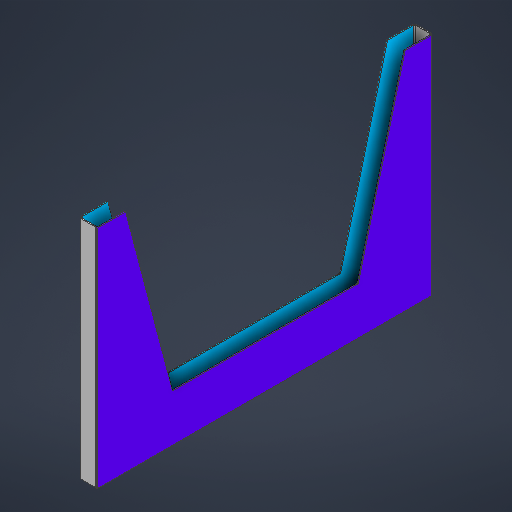
# Autodesk Inventor part: Div_Big
Saved by Autodesk Inventor 2025.1 (Build 291241000, 241)
## iProperties
Created: 2024-09-26
Part Number: Div_Big
Material: Generic
Document SubType Name: Sheet Metal
Designer: rocky
Density: 1 g/cm^3
Sheet Metal Rule: Default
Appearance: Default
Flat Pattern Width: 60.96 cm
Flat Pattern Length: 189.571 cm
Flat Pattern Area: 11556.3 cm^2
Sheet Metal Width: 24.000 in
Sheet Metal Length: 74.634 in
Sheet Metal Area: 1791.223 in^2
Author: rocky
Autodesk Inventor part; units mm, degrees
ref_plane "YZ Plane" through (0, 0, 0) normal (1, 0, 0) x (0, 1, 0)
ref_plane "XZ Plane" through (0, 0, 0) normal (0, 1, 0) x (-1, 0, 0)
ref_plane "XY Plane" through (0, 0, 0) normal (0, 0, 1) x (1, 0, 0)
sketch "Sketch1" plane through (0, 0, 0) normal (1, 0, 0) x (0, 1, 0)
  line L0 (0, 0) -> (609.6, 0)
  line L1 (609.6, 0) -> (609.6, -908.05)
  line L2 (609.6, -908.05) -> (0, -908.05)
  line L3 (0, -908.05) -> (0, 0)
  line L4 (127, 0) -> (127, -908.05)
  line L5 (609.6, 0) -> (127, -127)
  line L6 (609.6, -908.05) -> (127, -781.05)
  line L7 (609.6, -76.2) -> (127, -203.2)
  line L8 (609.6, -831.85) -> (127, -704.85)
  dimension "d0" = 609.6
  dimension "d1" = 908.05
  dimension "d2" = 127
  dimension "d3" = 127
  dimension "d4" = 127
  dimension "d6" = 76.2
  dimension "d7" = 76.2
  measures "d0" distance of L1.end L2.end
  measures "d1" distance of L0.end L1.end
  measures "d2" distance between parallel lines of L3 L4
  measures "d3" distance from line of L0 L5.end
  measures "d4" distance from line of L2 L6.end
  measures "d6" distance of L0.end L7.start
  measures "d7" distance from line of L2 L8.start
extrude "Plate1" add sketch "Sketch1" along normal blind 3.048 contours L0 L4 L2 L3 | L0 L5 L4 | L1 L7 L4 L5 | L4 L6 L2 | L6 L4 L8 L1
sketch "Sketch2" plane through (0, 609.6, -905.002) normal (0, 0, -1) x (-1, 0, 0)
  line L0 (0, -609.6) -> (0, 0)
  line L1 (0, 0) -> (-50.8, 0)
  line L2 (-50.8, 0) -> (-50.8, -609.6)
  line L3 (-50.8, -609.6) -> (0, -609.6)
  constraints: 6 end point, 1 horizontal, 1 perpendicular, 1 vertical
edge flange "Flange1" height 50.8 angle 90 thickness 3.048 bend radius 3.048 thickness toward (0, 0, -1) relief straight relief width 3.048 relief depth 1.524 edges at (3.048, 304.8, -908.05) wall of the first edge with corners at (0, 0, -905.002) (0, 609.6, -905.002) (50.8, 609.6, -905.002) (50.8, 0, -905.002)
bend "Bend1"
corner "Corner1"
sketch "Sketch3" plane through (47.752, 609.6, -908.05) normal (1, 0, 0) x (0, 1, 0)
  line L0 (-609.6, 0) -> (0, 0)
  line L1 (0, 0) -> (0, 939.8)
  line L2 (0, 939.8) -> (-609.6, 939.8)
  line L3 (-609.6, 939.8) -> (-609.6, 0)
  constraints: 6 end point, 1 horizontal, 1 perpendicular, 1 vertical
edge flange "Flange2" height 939.8 angle 90 thickness 3.048 bend radius 3.048 thickness toward (1, 0, 0) relief straight relief width 3.048 relief depth 1.524 edges at (50.8, 304.8, -905.002) wall of the first edge with corners at (47.752, 0, -908.05) (47.752, 609.6, -908.05) (47.752, 609.6, 31.75) (47.752, 0, 31.75)
bend "Bend2"
corner "Corner2"
sketch "Sketch4" plane through (0, 0, 0) normal (-1, 0, 0) x (0, 0, 1)
  line L0 (-901.954, 609.6) -> (-901.954, 0) projected
  line L1 (0, 0) -> (-901.954, 0) projected
  line L2 (0, 609.6) -> (0, 0) projected
  line L3 (-76.2, 609.6) -> (0, 609.6) projected
  line L4 (-203.2, 127) -> (-76.2, 609.6) projected
  line L5 (-704.85, 127) -> (-203.2, 127) projected
  line L6 (-831.85, 609.6) -> (-704.85, 127) projected
  line L7 (-901.954, 609.6) -> (-831.85, 609.6) projected
  line L8 (-908.05, 0) -> (-908.05, 609.6) projected
  line L9 (-901.954, 609.6) -> (-908.05, 609.6) projected
  line L10 (-908.05, 0) -> (-901.954, 0) projected
  line L11 (-908.05, 0) -> (-908.05, 609.6) projected
  line L12 (-901.954, 0) -> (-908.05, 0) projected
  line L13 (-901.954, 609.6) -> (-901.954, 0) projected
  line L14 (-908.05, 609.6) -> (-901.954, 609.6) projected
extrude "Extrusion1" cut sketch "Sketch4" against normal blind 76.2 keep common part
sketch "Sketch5" plane through (0, 0, -3.048) normal (0, 0, 1) x (1, 0, 0)
  line L0 (0, 609.6) -> (0, 0)
  line L1 (0, 0) -> (44.704, 0)
  line L2 (44.704, 0) -> (44.704, 609.6)
  line L3 (44.704, 609.6) -> (0, 609.6)
  constraints: 6 end point, 1 horizontal, 1 perpendicular, 1 vertical
edge flange "Flange3" height 44.704 angle 90 thickness 3.048 bend radius 3.048 thickness toward (0, 0, 1) relief straight relief width 3.048 relief depth 1.524 edges at (3.048, 304.8, 0) wall of the first edge with corners at (0, 609.6, -3.048) (0, 0, -3.048) (44.704, 0, -3.048) (44.704, 609.6, -3.048)
bend "Bend3"
corner "Corner3"
equation "\"d8\" = Thickness"
equation "\"d9\" = BendReliefWidth"
equation "\"d10\" = BendReliefDepth"
equation "\"d11\" = MinimumRemnant"
equation "\"d12\" = TransitionRadius"
equation "\"d15\" = BendRadius"
equation "\"d16\" = CornerReliefSize"
equation "\"d17\" = GapSize"
equation "\"d18\" = JacobiRadiusSize"
equation "\"d19\" = BendReliefWidth"
equation "\"d20\" = BendReliefDepth"
equation "\"d21\" = MinimumRemnant"
equation "\"d22\" = TransitionRadius"
equation "\"d25\" = BendRadius"
equation "\"d26\" = CornerReliefSize"
equation "\"d27\" = GapSize"
equation "\"d28\" = JacobiRadiusSize"
equation "\"d31\" = BendReliefWidth"
equation "\"d32\" = BendReliefDepth"
equation "\"d33\" = MinimumRemnant"
equation "\"d34\" = TransitionRadius"
equation "\"d37\" = BendRadius"
equation "\"d38\" = CornerReliefSize"
equation "\"d39\" = GapSize"
equation "\"d40\" = JacobiRadiusSize"
equation "\"BendRadius\" = Thickness"
equation "\"BendReliefWidth\" = Thickness"
equation "\"BendReliefDepth\" = 0.5 * Thickness"
equation "\"CornerReliefSize\" = 4 * Thickness"
equation "\"MinimumRemnant\" = 2 * Thickness"
equation "\"TransitionRadius\" = BendRadius"
equation "\"JacobiRadiusSize\" = BendRadius"
equation "\"GapSize\" = Thickness"
equation "\"Thickness\" = 3.048"
body "Solid1"
